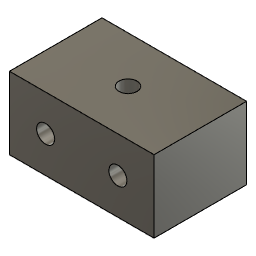
BearingTensionerBlock v13 (Autodesk Fusion 360 archive; units mm, degrees)
design "BearingTensionerBlock" references "tormach 770mx"
Autodesk Fusion 360 part; units mm, degrees
sketch "Sketch1" plane through (0, 0, 0) normal (0, 1, 0) x (1, 0, 0)
  line L0 (0, 0) -> (20, 0)
  line L1 (20, 0) -> (20, -12.8)
  line L2 (20, -12.8) -> (0, -12.8)
  line L3 (0, -12.8) -> (0, 0)
  dimension "d1" = 20
  dimension "d2" = 12.8
  constraint horizontal L0
  constraint vertical L1
  constraint horizontal L2
  constraint vertical L3
  constraint coincident L0.start L3.end
  measures "d1" distance of L0.start L0.end
  measures "d2" distance of L0.start L2.end
extrude "Extrude1" add sketch "Sketch1" along normal blind 10
sketch "Sketch2" plane through (0, 10, 0) normal (0, 1, 0) x (-1, 0, 0)
  line L0 (0, 12.8) -> (-20, 12.8)
  line L1 (-20, 12.8) -> (-20, 0)
  line L2 (-20, 0) -> (0, 0)
  line L3 (0, 0) -> (0, 12.8)
  line L4 (-10, 0) -> (-10, 12.8) construction
  line L5 (0, 6.4) -> (-20, 6.4) construction
  point P0 (-10, 6.4)
  constraint midpoint L2 L4.start
  constraint midpoint L0 L4.end
  constraint midpoint L3 L5.start
  constraint midpoint L1 L5.end
  constraint midpoint L4 P0
hole "Hole1" at (10, 10, 6.4) direction (0, -1, 0) diameter 2.5 end through all
sketch "Sketch3" plane through (0, 0, 12.8) normal (0, 0, 1) x (1, 0, 0)
  line L0 (0, 0) -> (20, 0)
  line L1 (20, 0) -> (20, 10)
  line L2 (20, 10) -> (0, 10)
  line L3 (0, 10) -> (0, 0)
  line L4 (0, 5) -> (20, 5) construction
  line L5 (5, 2.6) -> (5, 7.2) construction
  line L6 (15, 2.6) -> (15, 7.2) construction
  point P0 (5, 5)
  point P1 (15, 5)
  dimension "d8" = 10
  dimension "d9" = 5
  dimension "d16" = 5
  constraint coincident L3 L4.start
  constraint coincident L1 L4.end
  constraint perpendicular L1 L4
  constraint perpendicular L4 L5
  constraint perpendicular L4 L6
  constraint coincident L4 P0
  constraint coincident L5 P0
  constraint coincident L6 P1
  constraint coincident L4 P1
  measures "d8" distance of L5.start L6.start
  measures "d9" distance of L3 L5.start
  measures "d16" distance of L2 L4
hole "Hole4" at (5, 5, 12.8) direction (0, 0, -1) diameter 2.5 end through all
hole "Hole5" at (15, 5, 12.8) direction (0, 0, -1) diameter 2.5 end through all
